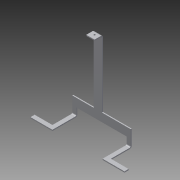
# Autodesk Inventor part: Puller Mechanism
Saved by Autodesk Inventor 2013 (Build 170138000, 138)
## iProperties
Created: 2013-01-28
Part Number: Puller Mechanism
Material: Aluminum 6061
Document SubType Name: Sheet Metal
Designer: Andrew Toennies
Density: 2.71 g/cm^3
Sheet Metal Rule: Default
Mass: 120.38 g
Surface Area: 326.479 cm^2
Volume: 44.4206 cm^3
Author: Andrew Toennies
Autodesk Inventor part; units mm, degrees
ref_plane "YZ Plane" through (0, 0, 0) normal (1, 0, 0) x (0, 1, 0)
ref_plane "XZ Plane" through (0, 0, 0) normal (0, 1, 0) x (-1, 0, 0)
ref_plane "XY Plane" through (0, 0, 0) normal (0, 0, 1) x (1, 0, 0)
sketch "Sketch5" plane through (-64.77, -47.625, 76.2) normal (0, 1, 0) x (1, 0, 0)
  line L0 (0, 0) -> (0, 69.85)
  line L1 (177.8, 69.85) -> (165.1, 69.85)
  line L2 (165.1, 0) -> (165.1, 69.85)
  line L3 (165.1, 0) -> (177.8, 0)
  line L4 (177.8, 0) -> (177.8, 69.85)
  line L5 (0, 0) -> (-53.975, 0)
  line L6 (-53.975, 0) -> (-53.975, 12.7)
  line L7 (-53.975, 12.7) -> (0, 12.7)
  line L8 (177.8, 0) -> (231.775, 0)
  line L9 (231.775, 0) -> (231.775, 12.7)
  line L10 (231.775, 12.7) -> (177.8, 12.7)
  point P0 (64.77, 76.2)
  dimension "d37" = 53.975
  dimension "d38" = 12.7
  dimension "d39" = 53.975
  dimension "d40" = 12.7
  measures "d37" distance of L0.start L5.end
  measures "d38" distance of L5.end L6.end
  measures "d39" distance of L3.end L8.end
  measures "d40" distance of L8.end L9.end
sketch "Sketch1" plane through (0, 0, 0) normal (0, 0, 1) x (1, 0, 0)
  line L0 (0, 0) -> (0, 203.2)
  line L1 (0, 203.2) -> (25.4, 203.2)
  line L2 (25.4, 203.2) -> (25.4, 0)
  line L3 (25.4, 0) -> (113.03, 0)
  line L4 (113.03, 0) -> (113.03, -25.4)
  line L5 (113.03, -25.4) -> (113.03, -50.8)
  line L6 (113.03, -50.8) -> (100.33, -50.8)
  line L7 (100.33, -50.8) -> (100.33, -25.4)
  line L8 (100.33, -25.4) -> (-52.07, -25.4)
  line L9 (-52.07, -25.4) -> (-52.07, -50.8)
  line L10 (-52.07, -50.8) -> (-64.77, -50.8)
  line L11 (-64.77, -50.8) -> (-64.77, 0)
  line L12 (-64.77, 0) -> (0, 0)
  dimension "d0" = 203.2
  dimension "d1" = 25.4
  dimension "d2" = 87.63
  dimension "d3" = 25.4
  dimension "d4" = 25.4
  dimension "d5" = 12.7
  dimension "d6" = 25.4
  dimension "d7" = 12.7
  dimension "d8" = 64.77
  dimension "d9" = 25.4
  dimension "d10" = 25.4
  measures "d0" distance of L0.start L0.end
  measures "d1" distance of L0.end L1.end
  measures "d2" distance of L2.end L3.end
  measures "d3" distance of L3.end L4.end
  measures "d4" distance of L4.end L5.end
  measures "d5" distance of L5.end L6.end
  measures "d6" distance of L8.end L9.end
  measures "d7" distance of L9.end L10.end
  measures "d8" distance of L11.end L0.start
  measures "d9" distance between parallel lines of L8 L3
  measures "d10" distance between parallel lines of L8 L12
extrude "Plate1" add sketch "Sketch1" along normal blind 3.175
sketch "Sketch2" plane through (-52.07, -47.625, 0) normal (0, -1, 0) x (1, 0, 0)
  line L0 (-12.7, 0) -> (0, 0)
  line L1 (0, 0) -> (0, 76.2)
  line L2 (0, 76.2) -> (-12.7, 76.2)
  line L3 (-12.7, 76.2) -> (-12.7, 0)
  constraints: 6 end point, 1 horizontal, 1 perpendicular, 1 vertical
edge flange "Flange1" height 76.2 angle 90 thickness 3.175 bend radius 3.175 thickness toward (0, -1, 0) relief straight relief width 3.175 relief depth 1.5875 corner gap 3.175 corner form 0 edges at (-58.42, -50.8, 3.175) (106.68, -50.8, 3.175) wall of the first edge with corners at (-64.77, -47.625, 0) (-52.07, -47.625, 0) (-52.07, -47.625, 76.2) (-64.77, -47.625, 76.2)
bend "Bend1"
corner "Corner1"
sketch "Sketch3" plane through (0, 200.025, 0) normal (0, 1, 0) x (-1, 0, 0)
  line L0 (-25.4, 0) -> (0, 0)
  line L1 (0, 0) -> (0, 25.4)
  line L2 (0, 25.4) -> (-25.4, 25.4)
  line L3 (-25.4, 25.4) -> (-25.4, 0)
  constraints: 6 end point, 1 horizontal, 1 perpendicular, 1 vertical
edge flange "Flange2" height 25.4 angle 90 thickness 3.175 bend radius 3.175 thickness toward (0, 1, 0) relief straight relief width 3.175 relief depth 1.5875 edges at (12.7, 203.2, 3.175) wall of the first edge with corners at (25.4, 200.025, 0) (0, 200.025, 0) (0, 200.025, 25.4) (25.4, 200.025, 25.4)
bend "Bend2"
corner "Corner2"
sketch "Sketch4" plane through (0, 203.2, 25.4) normal (0, 1, 0) x (1, 0, 0)
  line L0 (25.4, 0) -> (0, 0) projected
  line L1 (25.4, 19.05) -> (25.4, 0) projected
  circle A0 centre (12.7, 12.7) radius 2.413
  point P0 (0, 25.4)
  dimension "d32" = 4.826
  dimension "d33" = 12.7
  dimension "d34" = 12.7
  constraints: 1 centre point
  measures "d32" diameter of A0
  measures "d33" distance from line of L1 A0.centre
  measures "d34" distance from line of L0 A0.centre
extrude "Cut1" cut sketch "Sketch4" against normal blind 3.175
sheet face with bend "Face2" sketch "Sketch5" thickness 3.175 toward (0, -1, 0) bend radius 3.175 relief straight relief width 3.175 relief depth 1.5875 contours L5 L6 L7 L0 | L10 L9 L8 L4
bend "Bend3"
equation "\"d35\" = Thickness"
equation "\"d12\" = BendReliefWidth"
equation "\"d13\" = BendReliefDepth"
equation "\"d14\" = MinimumRemnant"
equation "\"d15\" = BendRadius"
equation "\"d18\" = BendRadius"
equation "\"d19\" = CornerReliefSize"
equation "\"d20\" = GapSize"
equation "\"d21\" = JacobiRadiusSize"
equation "\"d22\" = BendReliefWidth"
equation "\"d23\" = BendReliefDepth"
equation "\"d24\" = MinimumRemnant"
equation "\"d25\" = BendRadius"
equation "\"d28\" = BendRadius"
equation "\"d29\" = CornerReliefSize"
equation "\"d30\" = GapSize"
equation "\"d31\" = JacobiRadiusSize"
equation "\"d41\" = BendRadius"
equation "\"d42\" = BendReliefWidth"
equation "\"d44\" = MinimumRemnant"
equation "\"d43\" = BendReliefDepth"
equation "\"d45\" = BendRadius"
equation "\"BendRadius\" = Thickness"
equation "\"BendReliefWidth\" = Thickness"
equation "\"BendReliefDepth\" = 0.5 * Thickness"
equation "\"CornerReliefSize\" = 4 * Thickness"
equation "\"MinimumRemnant\" = 2 * Thickness"
equation "\"TransitionRadius\" = BendRadius"
equation "\"JacobiRadiusSize\" = BendRadius"
equation "\"GapSize\" = Thickness"
equation "\"d11\" = BendRadius"
equation "\"Thickness\" = 3.175"
body "Solid1"
